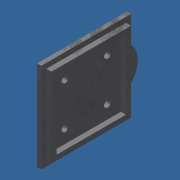
# Autodesk Inventor part: Modul Deckel
Saved by Autodesk Inventor 2018.2 (Build 222227000, 227)
## iProperties
Created: 2018-10-15
Part Number: Modul Deckel
Material: Kst - PVC (rigid/black)
Document SubType Name: Modeling
Designer: N.Grubert
Density: 1.38 g/cm^3
Appearance: Glatt - Mittelgrau
Fläche: 0 cm²
Gewicht: 0 g
Material: geeigneten Werkstoff auswählen !
Dateiname: P:\INVENTOR\Inventor 2018\Templates\ILT\Norm.ipt
Bez_eng: bolt
Bez_french: boulon
Author: N.Grubert
Autodesk Inventor part; units mm, degrees
ref_plane "YZ Plane" through (0, 0, 0) normal (1, 0, 0) x (0, 1, 0)
ref_plane "XZ Plane" through (0, 0, 0) normal (0, 1, 0) x (-1, 0, 0)
ref_plane "XY Plane" through (0, 0, 0) normal (0, 0, 1) x (1, 0, 0)
sketch "Skizze4" plane through (0, 0, 0) normal (1, 0, 0) x (0, 1, 0)
  line L0 (26.5, 26.5) -> (-26.5, 26.5)
  line L1 (-26.5, 26.5) -> (-26.5, -26.5)
  line L2 (-26.5, -26.5) -> (26.5, -26.5)
  line L3 (26.5, -26.5) -> (26.5, 26.5)
  line L4 (0, -37.1) -> (0, 37.1) construction
  line L5 (-37.1, 0) -> (37.1, 0) construction
  dimension "d18" = 53
  dimension "d19" = 53
  constraints: 8 end point, 3 parallel, 1 horizontal, 1 perpendicular, 2 other
  measures "d18" distance between parallel lines of L2 L0
  measures "d19" distance between parallel lines of L3 L1
extrude "Extrusion2" add sketch "Skizze4" along normal blind 2.5
sketch "Skizze5" plane through (2.5, 0, 0) normal (1, 0, 0) x (0, 0, -1)
  line L0 (-26.5, -26.5) -> (26.5, -26.5) construction
  line L1 (26.5, -26.5) -> (26.5, 26.5) construction
  line L2 (26.5, 26.5) -> (-26.5, 26.5) construction
  line L3 (-26.5, 26.5) -> (-26.5, -26.5) construction
  line L4 (-23.5, 23.5) -> (23.5, 23.5)
  line L5 (23.5, 23.5) -> (23.5, -23.5)
  line L6 (23.5, -23.5) -> (-23.5, -23.5)
  line L7 (-23.5, -23.5) -> (-23.5, 23.5)
  line L8 (20.5, 20.5) -> (-20.5, 20.5)
  line L9 (-20.5, 20.5) -> (-20.5, -20.5)
  line L10 (-20.5, -20.5) -> (20.5, -20.5)
  line L11 (20.5, -20.5) -> (20.5, 20.5)
  point P0 (0, 0)
  dimension "d8" = 3
  dimension "d9" = 3
  constraints: 16 end point, 6 other
  measures "d8" distance between parallel lines of L2 L4
  measures "d9" distance between parallel lines of L4 L8
extrude "Extrusion3" add sketch "Skizze5" along normal blind 3
sketch "Skizze6" plane through (0, 0, 0) normal (-1, 0, 0) x (0, 0, 1)
  line L0 (26.5, 26.5) -> (-26.5, 26.5) construction
  line L1 (26.5, -26.5) -> (26.5, 26.5) construction
  line L2 (-26.5, 26.5) -> (-26.5, 0) construction
  line L3 (0, -5.395) -> (0, 39.3226) construction
  line L4 (-26.5, 26.5) -> (26.5, 26.5) projected
  arc A0 (10.7474, 26.5) -> (-8.8486, 26.5) centre (0.9494, 16.5) ccw
  point P0 (0, 0)
  dimension "d12" = 26.5
  dimension "d13" = 53
  dimension "d14" = 14
  dimension "d15" = 10
  constraints: 2 end point, 2 point on circle, 2 point on line, 1 centre point, 1 vertical
  measures "d12" distance between parallel lines of L3 L1
  measures "d13" distance of L0.start L0.end
  measures "d14" radius of A0
  measures "d15" distance from line of A0.centre L0
extrude "Extrusion4" add sketch "Skizze6" against normal up to surface (2.5 mm away)
sketch "Skizze7" plane through (0, 0, 0) normal (-1, 0, 0) x (0, 0, 1)
  point P0 (0, 0)
  point P1 (-12.5, 12.5)
  point P2 (12.5, 12.5)
  point P3 (12.5, -12.5)
  point P4 (-12.5, -12.5)
  constraints: 4 other
hole "Bohrung1" at (0, 12.5, -12.5) at (0, 12.5, 12.5) at (0, -12.5, 12.5) at (0, -12.5, -12.5) direction (1, 0, 0) diameter 4 end through all
chamfer "Fase1" distance 2 angle 45 4 edges at (0, -12.5, -14.5) (0, 12.5, -14.5) (0, 12.5, 10.5) (0, -12.5, 10.5)
equation "\"d19\" = d18"
equation "\"d12\" = 0.5 * d13"
